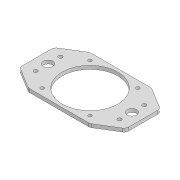
# Autodesk Inventor part: Suporte_inferior_menor
Saved by Autodesk Inventor 2020 (Build 240168000, 168)
## iProperties
Created: 2022-07-20
Part Number: Suporte_inferior_menor
Material: Genérico
Document SubType Name: Modeling
Designer: gabri
Density: 1 g/cm^3
Appearance: Padrão
Author: gabri
Autodesk Inventor part; units mm, degrees
ref_plane "YZ Plane" through (0, 0, 0) normal (1, 0, 0) x (0, 1, 0)
ref_plane "XZ Plane" through (0, 0, 0) normal (0, 1, 0) x (-1, 0, 0)
ref_plane "XY Plane" through (0, 0, 0) normal (0, 0, 1) x (1, 0, 0)
sketch "Esboço1" plane through (0, 0, 0) normal (0, 1, 0) x (-1, 0, 0)
  circle A0 centre (0, 0) radius 32.5
  line L0 (0, 0) -> (36, 0)
  line L1 (36, 0) -> (36, -36)
  line L2 (34.3118, -36) -> (0, -36)
  line L3 (0, -36) -> (0, 0)
  circle A1 centre (28, -28) radius 2
  circle A2 centre (49.1, 0) radius 5.5
  circle A3 centre (49.1, -14.5) radius 2.25
  line L4 (62.1814, 0) -> (62.1814, -16.635)
  line L5 (59.3102, -21.7547) -> (37.4405, -35.1197)
  line L6 (62.1814, 0) -> (36, 0)
  arc A4 (59.3102, -21.7547) -> (62.1814, -16.635) centre (56.1814, -16.635) ccw
  arc A5 (34.3118, -36) -> (37.4405, -35.1197) centre (34.3118, -30) ccw
  point P0 (32.5, 0)
  point P1 (0, -32.5)
  point P2 (62.1814, -20)
  point P3 (36, -35.7576)
  point P4 (54.6, 0)
  point P5 (43.6, 0)
  dimension "d0" = 65
  dimension "d1" = 36
  dimension "d2" = 36
  dimension "d4" = 4
  dimension "d9" = 11
  dimension "d10" = 13.1
  dimension "d11" = 4.5
  dimension "d12" = 14.5
  dimension "d13" = 20
  dimension "d14" = 6
  dimension "d15" = 6
  constraints: 14 end point, 6 centre point, 4 point on circle, 4 point on line, 4 tangent, 2 horizontal, 2 parallel, 1 coincident, 1 equal radius, 1 perpendicular, 1 vertical
  measures "d0" diameter of A0
  measures "d1" distance of L1.end L2.end
  measures "d2" distance of L1.end L0.end
  measures "d4" diameter of A1
  measures "d9" diameter of A2
  measures "d10" distance from line of A2.centre L1
  measures "d11" diameter of A3
  measures "d12" distance of A3.centre A2.centre
  measures "d13" distance of L4.start point (62.181, -20)
  measures "d14" radius of A4
  measures "d15" radius of A5
extrude "Extrusão1" add sketch "Esboço1" along normal blind 4 contours L0 L1 A5 L2 L3 A0 | L6 A2 L4 A4 L5 A5 L1
mirror "Espelhamento1" about plane through (0, 0, -32.5) normal (1, 0, 0) of "Extrusão1"
mirror "Espelhamento3" about plane through (43.6, 0, 0) normal (0, 0, 1) of "Extrusão1", "Espelhamento1"
